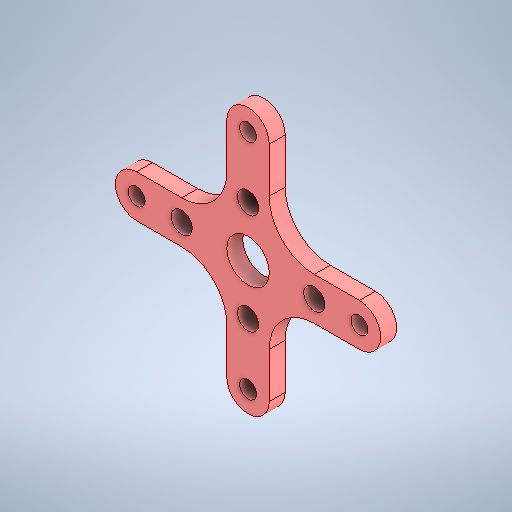
# Autodesk Inventor part: ACOPLE
Saved by Autodesk Inventor 2025.3 (Build 293356030, 356C)
## iProperties
Created: 2025-07-11
Part Number: ACOPLE
Material: Generic
Document SubType Name: Modeling
Designer: jv
Density: 1 g/cm^3
Appearance: Default(1)
Author: jv
Autodesk Inventor part; units mm, degrees
ref_plane "YZ Plane" through (0, 0, 0) normal (1, 0, 0) x (0, 1, 0)
ref_plane "XZ Plane" through (0, 0, 0) normal (0, 1, 0) x (-1, 0, 0)
ref_plane "XY Plane" through (0, 0, 0) normal (0, 0, 1) x (1, 0, 0)
sketch "Sketch1" plane through (0, 0, 0) normal (0, 0, 1) x (1, 0, 0)
  line L0 (-4, 25) -> (4, 25)
  line L1 (4, 25) -> (4, -25)
  line L2 (4, -25) -> (-4, -25)
  line L3 (-4, -25) -> (-4, 25)
  circle A0 centre (12.5, 0) radius 2
  circle A1 centre (-12.5, 0) radius 2
  circle A2 centre (21, 0) radius 1.6
  circle A3 centre (0, 21) radius 1.6
  circle A4 centre (-21, 0) radius 1.6
  circle A5 centre (0, -21) radius 1.6
  line L4 (-25, -4) -> (-25, 4)
  line L5 (-25, 4) -> (25, 4)
  line L6 (25, -4) -> (-25, -4)
  line L7 (25, 4) -> (25, -4)
  circle A6 centre (0, 21) radius 4
  circle A7 centre (21, 0) radius 4
  circle A8 centre (-21, 0) radius 4
  circle A9 centre (0, -21) radius 4
  circle A10 centre (12.5, 12.5) radius 8.5
  circle A11 centre (-12.5, 12.5) radius 8.5
  circle A12 centre (-12.5, -12.5) radius 8.5
  circle A13 centre (12.5, -12.5) radius 8.5
  circle A14 centre (0, 0) radius 4
  circle A15 centre (0, 9.5) radius 2
  circle A16 centre (0, -9.5) radius 2
  point P0 (4, 0)
  point P1 (0, 25)
  point P2 (-25, 0)
  point P3 (0, 4)
  point P4 (12.5, 4)
  point P5 (4, 12.5)
  point P6 (4, 21)
  point P7 (-4, 21)
  point P8 (-4, 12.5)
  point P9 (-12.5, 4)
  point P10 (-21, 4)
  point P11 (-21, -4)
  point P12 (-12.5, -4)
  point P13 (-4, -12.5)
  point P14 (-4, -21)
  point P15 (4, -21)
  point P16 (4, -12.5)
  point P17 (12.5, -4)
  point P18 (21, -4)
  point P19 (21, 4)
  point P20 (4, 4)
  point P21 (4, -4)
  point P22 (-4, -4)
  point P23 (-4, 4)
  point P24 (0, 4)
  point P25 (0, -4)
  point P26 (-4, 0)
  dimension "d0" = 4
  dimension "d3" = 360
  dimension "d5" = 3.2
  dimension "d8" = 360
  dimension "d10" = 8
  dimension "d13" = 90
  dimension "d15" = 50
  dimension "d16" = 42
  dimension "d17" = 4
  dimension "d19" = 17
  dimension "d22" = 360
  dimension "d27" = 4
  dimension "d30" = 360
  dimension "d32" = 19
  dimension "d33" = 25
  constraints: 16 end point, 14 centre point, 5 coincident, 2 midpoint, 2 parallel, 2 tangent, 1 horizontal, 1 horizontal alignment, 1 perpendicular, 1 vertical alignment, 48 other
  measures "d0" diameter of A0
  measures "d5" diameter of A2
  measures "d10" distance of L1.end L2.end
  measures "d15" distance between parallel lines of L2 L0
  measures "d16" distance of A5.centre A3.centre
  measures "d17" distance of point (0, 25) point (0, 21)
  measures "d19" diameter of A10
  measures "d27" diameter of A15
  measures "d32" distance of A16.centre A15.centre
  measures "d33" distance of A0.centre A1.centre
extrude "Extrusion1" add sketch "Sketch1" along normal blind 3 contours A6 | A6 L1 L5 L3 | L3 L5 A11 | A10 L5 L1 | L5 A14 L3 | L3 L6 A8 L5 | L5 A7 L6 L1 | L1 A14 L5 | A14 L6 L3 | A8 | L1 L6 A14 | A7 | L6 L1 A9 L3 | L3 A12 L6 | L6 A13 L1 | A9
body "Solid1"
